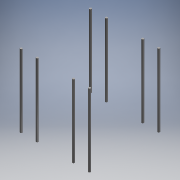
# Autodesk Inventor part: Gondola Poles
Saved by Autodesk Inventor 2018 (Build 220112000, 112)
## iProperties
Created: 2018-02-09
Part Number: Gondola Poles
Material: Steel, Alloy
Document SubType Name: Modeling
Designer: Joey
Density: 7.73 g/cm^3
Appearance: Semi-Polished
Author: Joey
Autodesk Inventor part; units mm, degrees
ref_plane "YZ Plane" through (0, 0, 0) normal (1, 0, 0) x (0, 1, 0)
ref_plane "XZ Plane" through (0, 0, 0) normal (0, 1, 0) x (-1, 0, 0)
ref_plane "XY Plane" through (0, 0, 0) normal (0, 0, 1) x (1, 0, 0)
sketch "Sketch1" plane through (0, 0, 0) normal (0, 1, 0) x (-1, 0, 0)
  circle A0 centre (850.9, -1016) radius 31.75
  line L0 (-914.4, 1066.8) -> (914.4, 1066.8) construction
  line L1 (914.4, 1066.8) -> (914.4, -1066.8) construction
  line L2 (914.4, -1066.8) -> (-914.4, -1066.8) construction
  line L3 (-914.4, -1066.8) -> (-914.4, 1066.8) construction
  line L4 (-914.4, 1066.8) -> (914.4, -1066.8) construction
  line L5 (914.4, 1066.8) -> (-914.4, -1066.8) construction
  circle A1 centre (381, -1016) radius 31.75
  circle A2 centre (850.9, 1016) radius 31.75
  circle A3 centre (-1155.7, -1016) radius 31.75
  circle A4 centre (-1155.7, 1016) radius 31.75
  circle A5 centre (381, 1016) radius 31.75
  circle A6 centre (-685.8, -1016) radius 31.75
  circle A7 centre (-685.8, 1016) radius 31.75
  point P0 (0, 0)
  dimension "d0" = 63.5
  dimension "d1" = 1828.8
  dimension "d2" = 2133.6
  dimension "d3" = 50.8
  dimension "d4" = 63.5
  dimension "d5" = 63.5
  dimension "d6" = 533.4
  dimension "d7" = 50.8
  dimension "d10" = 2032
  dimension "d13" = 2006.6
  dimension "d18" = 2032
  dimension "d21" = 1066.8
  constraints: 12 end point, 8 centre point, 3 horizontal, 2 midpoint, 2 parallel, 2 vertical, 1 perpendicular, 12 other
  measures "d0" diameter of A0
  measures "d1" distance of L1.end L2.end
  measures "d2" distance of L0.end L1.end
  measures "d3" distance from line of L2 A0.centre
  measures "d4" distance from line of A0.centre L1
  measures "d5" diameter of A1
  measures "d6" distance from line of A1.centre L1
  measures "d7" distance from line of L2 A1.centre
  measures "d10" distance of A0.centre A2.centre
  measures "d13" distance of A0.centre A3.centre
  measures "d18" distance of A1.centre A5.centre
  measures "d21" distance of A1.centre A6.centre
extrude "Extrusion1" add sketch "Sketch1" along normal mid plane 2133.6
body "Solid1"
